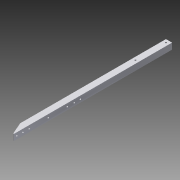
# Autodesk Inventor part: pickup arm 1x1 long
Saved by Autodesk Inventor 2015 (Build 190159000, 159)
## iProperties
Created: 2015-01-27
Part Number: pickup arm 1x1 long
Material: Aluminum 6061
Document SubType Name: Modeling
Designer: Admin
Density: 2.7 g/cm^3
Appearance: Aluminum - Flat
Author: Admin
Autodesk Inventor part; units mm, degrees
ref_plane "YZ Plane" through (0, 0, 0) normal (1, 0, 0) x (0, 1, 0)
ref_plane "XZ Plane" through (0, 0, 0) normal (0, 1, 0) x (-1, 0, 0)
ref_plane "XY Plane" through (0, 0, 0) normal (0, 0, 1) x (1, 0, 0)
sketch "Sketch1" plane through (0, 0, 0) normal (0, 0, 1) x (1, 0, 0)
  line L0 (0, 0) -> (25.4, 0)
  line L1 (25.4, 0) -> (25.4, 25.4)
  line L2 (25.4, 25.4) -> (0, 25.4)
  line L3 (0, 25.4) -> (0, 0)
  line L4 (3.175, 3.175) -> (22.225, 3.175)
  line L5 (22.225, 3.175) -> (22.225, 22.225)
  line L6 (22.225, 22.225) -> (3.175, 22.225)
  line L7 (3.175, 22.225) -> (3.175, 3.175)
  dimension "d0" = 25.4
  dimension "d1" = 25.4
  dimension "d2" = 19.05
  dimension "d3" = 19.05
  dimension "d4" = 3.175
  dimension "d5" = 3.175
  constraints: 16 end point, 4 parallel, 2 horizontal, 2 perpendicular
  measures "d0" distance of L2.end L1.end
  measures "d1" distance of L1.end L0.end
  measures "d2" distance of L6.end L5.end
  measures "d3" distance of L5.end L4.end
  measures "d4" distance between parallel lines of L0 L4
  measures "d5" distance between parallel lines of L3 L7
extrude "Extrusion1" add sketch "Sketch1" along normal blind 657.225
sketch "Sketch2" plane through (0, 25.4, 0) normal (0, 1, 0) x (1, 0, 0)
  line L0 (25.4, 0) -> (0, 0) projected
  line L1 (0, 0) -> (0, -657.225) projected
  point P0 (12.7, -12.7)
  point P1 (12.7, -139.7)
  dimension "d8" = 12.7
  dimension "d9" = 12.7
  dimension "d10" = 12.7
  dimension "d11" = 139.7
  measures "d8" distance from line of L0 point (12.7, -12.7)
  measures "d9" distance from line of L1 point (12.7, -12.7)
  measures "d10" distance from line of L1 point (12.7, -139.7)
  measures "d11" distance from line of L0 point (12.7, -139.7)
hole "Hole1" at (12.7, 25.4, 12.7) at (12.7, 25.4, 139.7) direction (0, -1, 0) diameter 6.35 end through all
sketch "Sketch3" plane through (0, 0, 0) normal (-1, 0, 0) x (0, 0, 1)
  line L0 (0, 0) -> (657.225, 0) projected
  line L1 (657.225, 25.4) -> (657.225, 0) projected
  point P0 (644.525, 12.7)
  point P1 (619.125, 12.7)
  point P2 (406.4, 12.7)
  point P3 (381, 12.7)
  dimension "d19" = 12.7
  dimension "d20" = 12.7
  dimension "d21" = 12.7
  dimension "d22" = 25.4
  dimension "d23" = 212.725
  dimension "d24" = 12.7
  dimension "d25" = 12.7
  dimension "d26" = 25.4
  measures "d19" distance from line of L1 point (644.525, 12.7)
  measures "d20" distance from line of L0 point (644.525, 12.7)
  measures "d21" distance from line of L0 point (619.125, 12.7)
  measures "d22" distance of point (644.525, 12.7) point (619.125, 12.7)
  measures "d23" distance of point (619.125, 12.7) point (406.4, 12.7)
  measures "d24" distance from line of L0 point (406.4, 12.7)
  measures "d25" distance from line of L0 point (381, 12.7)
  measures "d26" distance of point (381, 12.7) point (406.4, 12.7)
hole "Hole2" at (0, 12.7, 644.525) at (0, 12.7, 619.125) at (0, 12.7, 406.4) at (0, 12.7, 381) direction (1, 0, 0) diameter 6.35 end through all
sketch "Sketch5" plane through (0, 25.4, 0) normal (0, 1, 0) x (1, 0, 0)
  circle A0 centre (12.7, -12.7) radius 3.175 projected
  circle A1 centre (12.7, -139.7) radius 3.175 projected
  line L0 (25.4, 0) -> (0, 0) projected
  line L1 (0, 0) -> (0, -657.225) projected
  line L2 (25.4, -657.225) -> (0, -657.225) projected
  line L3 (25.4, 0) -> (25.4, -657.225) projected
  line L4 (0, -657.225) -> (22.225, -657.225)
  line L5 (22.225, -657.225) -> (3.175, -657.225) projected
  line L6 (0, -657.225) -> (0, -606.425)
  line L7 (0, 0) -> (0, -657.225) projected
  line L8 (0, -606.425) -> (22.225, -657.225)
  dimension "d37" = 22.225
  dimension "d38" = 50.8
  constraints: 6 end point, 1 collinear, 1 point on line
  measures "d37" distance of L1.end L4.end
  measures "d38" distance of L1.end L6.end
extrude "Extrusion3" cut sketch "Sketch5" against normal blind 25.4 contours L8 L2 L1
sketch "Sketch6" plane through (25.4, 0, 0) normal (1, 0, 0) x (0, 0, -1)
  line L0 (0, 25.4) -> (-657.225, 25.4) projected
  line L1 (-657.225, 0) -> (-657.225, 25.4) projected
  point P0 (-593.725, 12.7)
  point P1 (-514.35, 12.7)
  point P2 (-434.975, 12.7)
  dimension "d41" = 12.7
  dimension "d42" = 63.5
  dimension "d43" = 142.875
  dimension "d44" = 12.7
  dimension "d45" = 12.7
  dimension "d46" = 222.25
  measures "d41" distance from line of L0 point (-593.725, 12.7)
  measures "d42" distance from line of L1 point (-593.725, 12.7)
  measures "d43" distance from line of L1 point (-514.35, 12.7)
  measures "d44" distance from line of L0 point (-514.35, 12.7)
  measures "d45" distance from line of L0 point (-434.975, 12.7)
  measures "d46" distance from line of L1 point (-434.975, 12.7)
hole "Hole3" at (25.4, 12.7, 593.725) at (25.4, 12.7, 514.35) at (25.4, 12.7, 434.975) direction (-1, 0, 0) diameter 6.35 end through all
body "Solid1"
